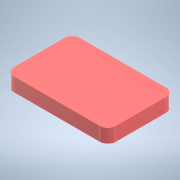
# Autodesk Inventor part: FactionSpecial_Nekro_XY
Saved by Autodesk Inventor 2021 (Build 250183000, 183)
## iProperties
Created: 2023-03-16
Part Number: FactionSpecial_Nekro_XY
Material: Paper
Document SubType Name: Modeling
Designer: Bradley
Density: 0.93 g/cm^3
Appearance: Smooth - Red
NekroLength: 16.400 mm
NekroWidth: 25.250 mm
Author: Bradley
Autodesk Inventor part; units mm, degrees
ref_plane "YZ Plane" through (0, 0, 0) normal (1, 0, 0) x (0, 1, 0)
ref_plane "XZ Plane" through (0, 0, 0) normal (0, 1, 0) x (-1, 0, 0)
ref_plane "XY Plane" through (0, 0, 0) normal (0, 0, 1) x (1, 0, 0)
sketch "Sketch1" plane through (0, 0, 0) normal (0, 1, 0) x (-1, 0, 0)
  line L0 (10.625, 8.2) -> (-10.625, 8.2)
  line L1 (-12.625, 6.2) -> (-12.625, -6.2)
  line L2 (-10.625, -8.2) -> (10.625, -8.2)
  line L3 (12.625, -6.2) -> (12.625, 6.2)
  line L4 (12.625, 8.2) -> (-12.625, -8.2) construction
  line L5 (-12.625, 8.2) -> (12.625, -8.2) construction
  arc A0 (12.625, 6.2) -> (10.625, 8.2) centre (10.625, 6.2) ccw
  arc A1 (10.625, -8.2) -> (12.625, -6.2) centre (10.625, -6.2) ccw
  arc A2 (-12.625, -6.2) -> (-10.625, -8.2) centre (-10.625, -6.2) ccw
  arc A3 (-10.625, 8.2) -> (-12.625, 6.2) centre (-10.625, 6.2) ccw
  point P0 (0, 0)
  dimension "d0" = 25.25
  dimension "d1" = 16.4
  dimension "d4" = 2
  constraints: 12 end point, 8 point on circle, 8 point on line, 8 tangent, 4 centre point, 3 equal radius, 2 midpoint, 2 parallel, 1 horizontal, 1 perpendicular
  measures "d0" distance of L5.end L4.end
  measures "d1" distance of L5.start L4.end
  measures "d4" radius of A0
extrude "Extrusion1" add sketch "Sketch1" along normal mid plane 3.4
equation "\"d0\" = NekroWidth"
equation "\"d1\" = NekroLength"
equation "\"NekroWidth\" = 25.25"
equation "\"NekroLength\" = 16.4"
body "Solid1"
